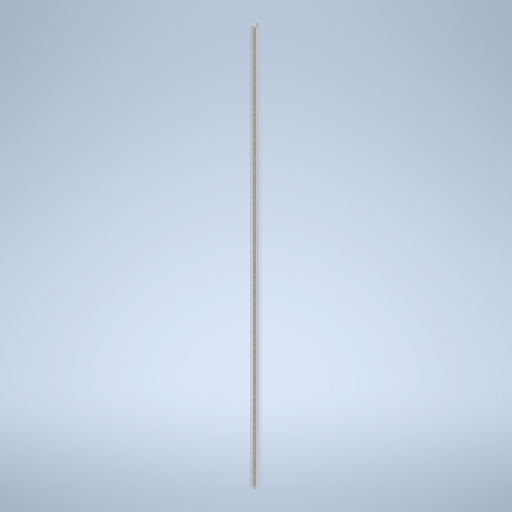
# Autodesk Inventor part: 96 tube
Saved by Autodesk Inventor 2024 (Build 280153000, 153)
## iProperties
Created: 2023-04-16
Part Number: 96 tube
Material: Aluminum 6061
Document SubType Name: Modeling
Designer: legom
Density: 2.7 g/cm^3
Appearance: Aluminum - Flat
Author: legom
Autodesk Inventor part; units mm, degrees
ref_plane "YZ Plane" through (0, 0, 0) normal (1, 0, 0) x (0, 1, 0)
ref_plane "XZ Plane" through (0, 0, 0) normal (0, 1, 0) x (-1, 0, 0)
ref_plane "XY Plane" through (0, 0, 0) normal (0, 0, 1) x (1, 0, 0)
sketch "Sketch4" plane through (0, 0, 0) normal (0, 1, 0) x (-1, 0, 0)
  line L0 (0, 0) -> (25.4, 0)
  line L1 (25.4, 0) -> (25.4, 25.4)
  line L2 (25.4, 25.4) -> (0, 25.4)
  line L3 (0, 25.4) -> (0, 0)
  line L4 (2.286, 2.286) -> (23.114, 2.286)
  line L5 (23.114, 2.286) -> (23.114, 23.114)
  line L6 (23.114, 23.114) -> (2.286, 23.114)
  line L7 (2.286, 23.114) -> (2.286, 2.286)
  dimension "d13" = 25.4
  dimension "d14" = 25.4
  dimension "d15" = 2.286
  constraints: 16 end point, 4 parallel, 2 perpendicular, 1 horizontal, 3 other
  measures "d13" distance of L2.end L1.end
  measures "d14" distance of L1.end L0.end
  measures "d15" distance between parallel lines of L3 L7
extrude "Extrusion2" add sketch "Sketch4" along normal blind 2387.6
sketch "Sketch5" plane through (0, 0, 25.4) normal (0, 0, 1) x (1, 0, 0)
  circle A0 centre (-12.7, 12.7) radius 2.5527
  line L0 (-25.4, 0) -> (0, 0) projected
  line L1 (-25.4, 0) -> (-25.4, 2387.6) projected
  dimension "d18" = 5.1054
  dimension "d19" = 12.7
  dimension "d20" = 12.7
  constraints: 1 centre point
  measures "d18" diameter of A0
  measures "d19" distance from line of L0 A0.centre
  measures "d20" distance from line of L1 A0.centre
extrude "Extrusion3" cut sketch "Sketch5" against normal through all
pattern_linear "Rectangular Pattern1" count 94 spacing 25.4 along (0, 1, 0) of "Extrusion3"
body "Solid2"
